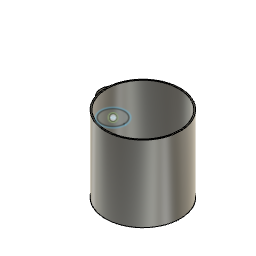
_well 3D prints.152b1785-663c-4be8-bdcb-cdfd87ff8bf2 (Autodesk Fusion 360 design; units mm, degrees)
Autodesk Fusion 360 part; units mm, degrees
sketch "Sketch1" plane through (0, 0, 0) normal (0, 0, 1) x (1, 0, 0)
  circle A0 centre (-67.4074, 43.4921) radius 10
  circle A1 centre (-67.4074, 43.4921) radius 1
  dimension "d1" = 20
  dimension "d2" = 2
  constraint concentric A0 A1
  measures "d1" diameter of A0
  measures "d2" diameter of A1
extrude "Extrude1" add sketch "Sketch1" along normal blind 15 makes body 1
sketch "Sketch2" plane through (0, 0, 0) normal (0, 0, 1) x (1, 0, 0)
  circle A0 centre (-67.4999, 43.4872) radius 9
  dimension "d5" = 18
  measures "d5" diameter of A0
extrude "Extrude2" cut sketch "Sketch2" along normal blind 14 bodies 1
sketch "Sketch3" plane through (0, 0, 0) normal (0, 1, 0) x (1, 0, 0)
sketch "Sketch4" plane through (0, 0, 0) normal (0, 0, 1) x (1, 0, 0)
  circle A0 centre (0, 0) radius 30
  circle A1 centre (-7.5952, 18.3974) radius 2.5
  circle A2 centre (-12.1351, -15.7763) radius 2.5
  circle A3 centre (19.7302, -2.6211) radius 2.5
  dimension "d8" = 60
  dimension "d9" = 5
  dimension "d11" = 360
  constraint coincident A0.centre origin
  measures "d8" diameter of A0
  measures "d9" diameter of A1
extrude "Extrude3" add sketch "Sketch4" along normal blind 1 separate body makes body 2
sketch "Sketch5" plane through (0, 0, 1) normal (0, 0, 1) x (-1, 0, 0)
  circle A0 centre (7.5952, -18.3974) radius 2.5
  circle A1 centre (-19.7302, 2.6211) radius 2.5
  circle A2 centre (12.1351, 15.7763) radius 2.5
  circle A3 centre (0, 0) radius 30
  circle A4 centre (0, 0) radius 29
  dimension "d14" = 58
  constraint coincident A3.centre A4.centre
  measures "d14" diameter of A4
extrude "Extrude4" add sketch "Sketch5" along normal blind 60 contours A3 bodies 2
